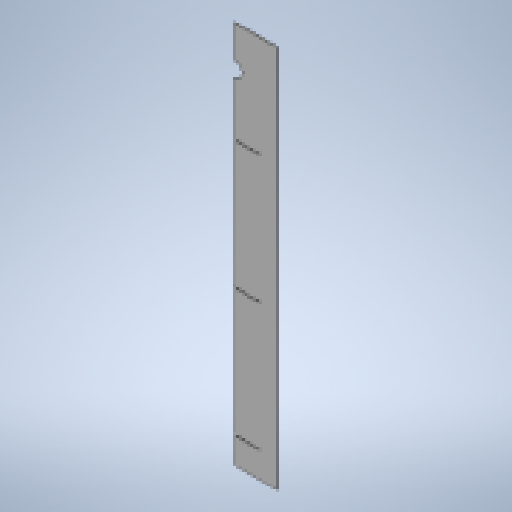
# Autodesk Inventor part: GBK 3114 stringer 2
Saved by Autodesk Inventor 2026 (Build 300175000, 175)
## iProperties
Created: 2026-05-07
Part Number: GBK 3114 stringer 2
Material: Steel
Document SubType Name: Sheet Metal
Designer: pokla
Mass: 8271.89 g
Surface Area: 5430.27 cm^2
Volume: 1053.74 cm^3
Density: 7.85 g/cm^3
Flat Pattern Width: 17.536 cm
Flat Pattern Length: 149 cm
Flat Pattern Area: 2612.86 cm^2
Sheet Metal Rule: По умолчанию_мм
Sheet Metal Width: 175,360 мм
Sheet Metal Length: 1490,000 мм
Sheet Metal Area: 261286,061 мм^2
Appearance: Default
Author: admin
Autodesk Inventor part; units mm, degrees
ref_plane "YZ Plane" through (0, 0, 0) normal (1, 0, 0) x (0, 1, 0)
ref_plane "XZ Plane" through (0, 0, 0) normal (0, 1, 0) x (-1, 0, 0)
ref_plane "XY Plane" through (0, 0, 0) normal (0, 0, 1) x (1, 0, 0)
sketch "Sketch1" plane through (0, 0, 0) normal (0, 0, 1) x (1, 0, 0)
  line L0 (0, 1490) -> (-175.3598, 1490)
  line L1 (-175.3598, 1490) -> (-175.3598, 0)
  line L2 (-175.3598, 0) -> (0, 0)
  line L3 (0, 0) -> (0, 1490)
  line L4 (-175.3598, 100) -> (-66, 100)
  line L5 (-66, 100) -> (-66, 105)
  line L6 (-66, 105) -> (-175.3598, 105)
  line L7 (-175.3598, 105) -> (-175.3598, 100)
  line L8 (-175.3598, 596.6667) -> (-66, 596.6667)
  line L9 (-66, 596.6667) -> (-66, 601.6667)
  line L10 (-66, 601.6667) -> (-175.3598, 601.6667)
  line L11 (-175.3598, 601.6667) -> (-175.3598, 596.6667)
  line L12 (-175.3598, 1093.3333) -> (-66, 1093.3333)
  line L13 (-66, 1093.3333) -> (-66, 1098.3333)
  line L14 (-66, 1098.3333) -> (-175.3598, 1098.3333)
  line L15 (-175.3598, 1098.3333) -> (-175.3598, 1093.3333)
  circle A0 centre (-175.3598, 1335) radius 30
  point P0 (-175.3598, 1098.3333)
  point P1 (-175.3598, 1093.3333)
  point P2 (-175.3598, 596.6667)
  point P3 (-175.3598, 1365)
  point P4 (-175.3598, 1305)
  dimension "d0" = 1490
  dimension "d1" = 175.3598
  dimension "d2" = 5
  dimension "d4" = 100
  dimension "d7" = 496.6667
  dimension "d23" = 66
  dimension "d29" = 60
  dimension "d30" = 1335
  measures "d0" distance of L1.end L0.end
  measures "d1" distance of L1.end L2.end
  measures "d2" distance of L4.end L5.end
  measures "d4" distance between parallel lines of L2 L4
  measures "d7" distance of L4.start L8.start
  measures "d23" distance between parallel lines of L3 L5
  measures "d29" diameter of A0
  measures "d30" distance from line of A0.centre L2
extrude "Plate1" add sketch "Sketch1" along normal blind 4 contours L3 L2 L1 L4 L5 L6 L8 L9 L10 L12 L13 L14 A0 L0
chamfer "Corner Chamfer1" distance 3 angle 45 6 edges at (-175.3598, 100, 2) (-175.3598, 105, 2) (-175.3598, 596.6667, 2) (-175.3598, 601.6667, 2) (-175.3598, 1098.3333, 2) (-175.3598, 1093.3333, 2)
equation "\"d0\" = Стрингер_длина"
equation "\"d1\" = стрингер_глубина_2"
equation "\"d2\" = паз_под_стрингер_толщина"
equation "\"d7\" = Шаг_шпангоутов"
equation "\"d23\" = паз_под_стрингер_глубина - Thickness"
equation "\"d29\" = 2 * радиус_выреза_под_сварку"
equation "\"d12\" = Thickness"
equation "\"BendRadius\" = Thickness"
equation "\"BendReliefWidth\" = Thickness"
equation "\"BendReliefDepth\" = 0.5 * Thickness"
equation "\"CornerReliefSize\" = 4 * Thickness"
equation "\"MinimumRemnant\" = 2 * Thickness"
equation "\"TransitionRadius\" = BendRadius"
equation "\"JacobiRadiusSize\" = BendRadius"
equation "\"GapSize\" = Thickness"
equation "\"Стрингер_длина\" = 1490"
equation "\"стрингер_глубина_2\" = 175.359772"
equation "\"паз_под_стрингер_толщина\" = 5"
equation "\"Шаг_шпангоутов\" = 496.666667"
equation "\"паз_под_стрингер_глубина\" = 70"
equation "\"Thickness\" = 4"
equation "\"радиус_выреза_под_сварку\" = 30"
body "Solid1"
